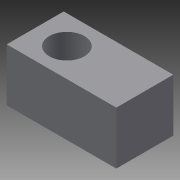
# Autodesk Inventor part: supporto_guide_10Z
Saved by Autodesk Inventor 2014 SP1 (Build 180222100, 222)
## iProperties
Created: 2015-04-08
Part Number: supporto_guide_10Z
Material: Generic
Document SubType Name: Modeling
Designer: Giorgio Nuzzo
Density: 1 g/cm^3
Appearance: Default
d0: 31,153 mm
d1: 16,200 mm
d2: 15,000 mm
d3: 0,00 deg
d5: 10,000 mm
d6: 9,000 mm
d7: 10,000 mm
d8: 0,00 deg
Author: Giorgio Nuzzo
Autodesk Inventor part; units mm, degrees
ref_plane "YZ Plane" through (0, 0, 0) normal (1, 0, 0) x (0, 1, 0)
ref_plane "XZ Plane" through (0, 0, 0) normal (0, 1, 0) x (-1, 0, 0)
ref_plane "XY Plane" through (0, 0, 0) normal (0, 0, 1) x (1, 0, 0)
sketch "Sketch1" plane through (0, 0, 0) normal (0, 0, 1) x (1, 0, 0)
  line L0 (-15.5765, 8.1) -> (15.5765, 8.1)
  line L1 (15.5765, 8.1) -> (15.5765, -8.1)
  line L2 (15.5765, -8.1) -> (-15.5765, -8.1)
  line L3 (-15.5765, -8.1) -> (-15.5765, 8.1)
  line L4 (0, 11.34) -> (0, -11.34) construction
  line L5 (-21.8071, 0) -> (21.8071, 0) construction
  point P0 (0, 0)
  dimension "d0" = 31.153
  dimension "d1" = 16.2
  constraints: 8 end point, 2 parallel, 1 horizontal, 1 perpendicular, 2 other
  measures "d0" distance of L0.start L0.end
  measures "d1" distance of L2.end L0.start
extrude "Extrusion1" add sketch "Sketch1" along normal blind 15
sketch "Sketch2" plane through (0, 0, 15) normal (0, 0, 1) x (1, 0, 0)
  line L0 (-15.5765, 8.1) -> (-15.5765, -8.1) projected
  circle A0 centre (-6.5765, 0) radius 5
  line L1 (-21.8071, 0) -> (21.8071, 0) construction
  point P0 (0, 0)
  dimension "d5" = 10
  dimension "d6" = 9
  constraints: 1 centre point, 1 point on line
  measures "d5" diameter of A0
  measures "d6" distance from line of L0 A0.centre
extrude "Extrusion2" cut sketch "Sketch2" against normal blind 10
body "Solid1"
